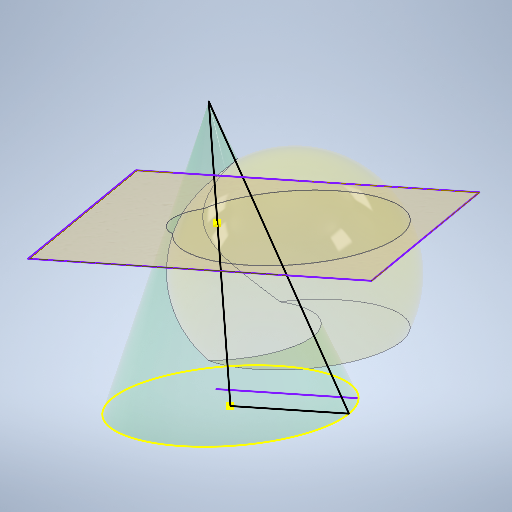
# Autodesk Inventor part: Комбинирование
Saved by Autodesk Inventor 2025 (Build 290162000, 162)
## iProperties
Created: 2024-11-18
Part Number: Комбинирование
Material: Типовые
Document SubType Name: Modeling
Designer: shoptick
Density: 1 g/cm^3
Appearance: Прозрачный — грифельно-синий
Author: shoptick
Autodesk Inventor part; units mm, degrees
ref_plane "YZ Plane" through (0, 0, 0) normal (1, 0, 0) x (0, 1, 0)
ref_plane "XY Plane" through (0, 0, 0) normal (0, 0, 1) x (1, 0, 0)
sketch "Эскиз1" plane through (0, 0, 0) normal (0, 0, 1) x (1, 0, 0)
  line L0 (0, 0) -> (40, 0)
  line L1 (0, 0) -> (0, 100)
  line L2 (0, 100) -> (40, 0)
  dimension "d0" = 40
  dimension "d1" = 100
  constraints: 6 end point, 1 horizontal, 1 vertical
  measures "d0" distance of L0.start L0.end
  measures "d1" distance of L0.start L1.end
revolve "Вращение1" add sketch "Эскиз1" angle 360 about axis through (0, 0, 0) along (0, 1, 0)
sketch "Эскиз2" plane through (0, 0, 0) normal (0, 0, 1) x (1, 0, 0)
  line L0 (40, 0) -> (-40, 0) projected
  arc A0 (59.641, 25) -> (25, 85) centre (25, 45) ccw
  line L1 (25, 25) -> (59.641, 25)
  line L2 (25, 25) -> (25, 85)
  point P0 (0, 0)
  dimension "d5" = 80
  dimension "d6" = 20
  constraints: 4 end point, 2 point on circle, 1 centre point, 1 horizontal, 1 vertical
  measures "d5" diameter of A0
  measures "d6" distance of A0.centre L1.start
revolve "Вращение2" add sketch "Эскиз2" angle 360 about axis through (25, 25, 0) along (0, 1, 0)
sketch "Эскиз3" plane through (0, 0, 0) normal (0, 1, 0) x (-1, 0, 0)
  line L0 (10.9603, -14.8081) -> (-37.158, -14.8081)
  circle A0 centre (0, 0) radius 40 projected
  constraints: 2 end point, 1 horizontal, 2 other
ref_plane "РабПлоскость1" through (0, 60, 0) normal (0, 1, 0) x (-1, 0, 0)
sketch "Эскиз4" plane through (0, 60, 0) normal (0, 1, 0) x (-1, 0, 0)
  line L0 (45.7608, -44.229) -> (-70.1729, -44.229)
  line L1 (-70.1729, -44.229) -> (-70.1729, 44.0375)
  line L2 (-70.1729, 44.0375) -> (45.7608, 44.0375)
  line L3 (45.7608, 44.0375) -> (45.7608, -44.229)
  point P0 (0, 0)
  constraints: 8 end point, 2 parallel, 1 horizontal, 1 perpendicular
extrude "Выдавливание1" add sketch "Эскиз4" along normal blind 0.1
